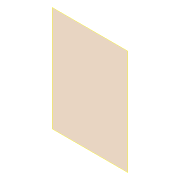
# Autodesk Inventor part: 30_Adapter_neje_LED
Saved by Autodesk Inventor 2019.4 (Build 234330000, 330)
## iProperties
Created: 2021-04-13
Part Number: 30_Adapter_neje_LED
Material: Generic
Document SubType Name: Modeling
Designer: diederichbenedict
Density: 1 g/cm^3
Appearance: Default
Author: diederichbenedict
Autodesk Inventor part; units mm, degrees
ref_plane "YZ Plane" through (0, 0, 0) normal (1, 0, 0) x (0, 1, 0)
ref_plane "XZ Plane" through (0, 0, 0) normal (0, 1, 0) x (-1, 0, 0)
ref_plane "XY Plane" through (0, 0, 0) normal (0, 0, 1) x (1, 0, 0)
ref_plane "Work Plane1" through (0, 0, 0) normal (0, 0, 1) x (1, 0, 0)
ref_plane "Work Plane2" through (0, 0, -24) normal (0, 0, 1) x (1, 0, 0)
sketch "Sketch1" plane through (0, 0, -24) normal (0, 0, 1) x (1, 0, 0)
  line L0 (-28.32, -15) -> (-28.32, -9.975) projected
  line L1 (-28.32, -3.975) -> (-28.32, 4.075) projected
  line L2 (-23.82, -15) -> (-28.32, -15) projected
  line L3 (-23.82, -15) -> (-23.52, -15)
  line L4 (-23.52, -15) -> (-23.82, -12.9669)
  line L5 (-23.82, -12.9669) -> (-18.8601, -12.9669)
  line L6 (-18.8601, -12.9669) -> (-18.8601, -18.9669)
  line L7 (-18.8601, -18.9669) -> (-92.6205, -18.9669)
  line L8 (-92.6205, -18.9669) -> (-92.6205, 137.182)
  line L9 (-92.6205, 137.182) -> (-83.4923, 137.182)
  line L10 (-83.4923, 137.182) -> (-83.4923, 6.5025)
  line L11 (-83.4923, 6.5025) -> (-28.32, 6.5025)
  line L12 (-28.32, -3.975) -> (-26.9128, -9.975)
  line L13 (-26.9128, -9.975) -> (-28.4348, -9.773)
  line L14 (-28.4348, -9.773) -> (-28.32, -10.5507)
  line L15 (-28.32, -10.5507) -> (-28.32, -15)
  line L16 (-28.32, -15) -> (-23.82, -15)
  line L17 (-28.32, 4.075) -> (-28.32, 4.2239)
  line L18 (-28.32, 4.2239) -> (-26.4709, 4.2239)
  line L19 (-26.4709, 4.2239) -> (-26.4709, 6.5025)
  line L20 (-26.4709, 6.5025) -> (-28.32, 6.5025)
  point P0 (0, 0)
  dimension "d0" = 0.3
  dimension "d1" = 6
  constraints: 36 end point, 9 perpendicular, 2 collinear, 2 parallel, 2 point on line, 1 horizontal, 1 vertical
  measures "d0" distance of L2.start L3.end
  measures "d1" distance of L5.end L6.end
extrude "Extrusion1" add sketch "Sketch1" along normal mid plane 20
fillet "Fillet1" radius 1 1 edges at (-26.9128, -9.975, -24)
chamfer "Chamfer1" distance 20 angle 45 2 edges at (-83.4923, 6.5025, -24) (-92.6205, -18.9669, -24)
sketch "Sketch2" plane through (-92.6205, 137.182, -34) normal (-1, 0, 0) x (0, 0, 1)
  line L0 (18.675, -27.877) -> (18.675, 6.063) projected
  line L1 (-16.4278, 9.4711) -> (-17.2496, 12.5384) projected
  line L2 (-17.2496, 12.5384) -> (-20.3169, 13.3602) projected
  line L3 (-20.3169, 13.3602) -> (-22.5622, 11.1149) projected
  line L4 (-22.5622, 11.1149) -> (-21.7404, 8.0476) projected
  line L5 (-21.7404, 8.0476) -> (-18.6731, 7.2258) projected
  line L6 (-18.6731, 7.2258) -> (-16.4278, 9.4711) projected
  line L7 (23.7269, -35.1742) -> (25.9722, -32.9289) projected
  line L8 (25.9722, -32.9289) -> (25.1504, -29.8616) projected
  line L9 (25.1504, -29.8616) -> (22.0831, -29.0398) projected
  line L10 (22.0831, -29.0398) -> (19.8378, -31.2851) projected
  line L11 (19.8378, -31.2851) -> (20.6596, -34.3524) projected
  line L12 (20.6596, -34.3524) -> (23.7269, -35.1742) projected
  circle A0 centre (16.005, 9.753) radius 2.475 projected
  circle A1 centre (-18.955, 3.393) radius 2.475 projected
  circle A2 centre (-12.595, -31.567) radius 2.475 projected
  circle A3 centre (22.365, -25.207) radius 2.475 projected
  circle A4 centre (22.365, 3.393) radius 2.475 projected
  circle A5 centre (16.005, -31.567) radius 2.475 projected
  circle A6 centre (-18.955, -25.207) radius 2.475 projected
  circle A7 centre (-12.595, 9.753) radius 2.475 projected
  arc A8 (-20.655, -19.707) -> (-17.255, -19.707) centre (-18.955, -19.707) ccw projected
  line L13 (-17.255, -19.707) -> (-17.255, -2.107) projected
  arc A9 (-17.255, -2.107) -> (-20.655, -2.107) centre (-18.955, -2.107) ccw projected
  line L14 (-20.655, -2.107) -> (-20.655, -19.707) projected
  arc A10 (20.665, -19.707) -> (24.065, -19.707) centre (22.365, -19.707) ccw projected
  line L15 (24.065, -19.707) -> (24.065, -2.107) projected
  arc A11 (24.065, -2.107) -> (20.665, -2.107) centre (22.365, -2.107) ccw projected
  line L16 (20.665, -2.107) -> (20.665, -19.707) projected
  arc A12 (10.505, -33.267) -> (10.505, -29.867) centre (10.505, -31.567) ccw projected
  line L17 (10.505, -29.867) -> (-7.095, -29.867) projected
  arc A13 (-7.095, -29.867) -> (-7.095, -33.267) centre (-7.095, -31.567) ccw projected
  line L18 (-7.095, -33.267) -> (10.505, -33.267) projected
  arc A14 (-7.095, 11.453) -> (-7.095, 8.053) centre (-7.095, 9.753) ccw projected
  line L19 (-7.095, 8.053) -> (10.505, 8.053) projected
  arc A15 (10.505, 8.053) -> (10.505, 11.453) centre (10.505, 9.753) ccw projected
  line L20 (10.505, 11.453) -> (-7.095, 11.453) projected
  line L21 (-15.265, -27.877) -> (18.675, -27.877) projected
  line L22 (18.675, -27.877) -> (18.675, 6.063) projected
  line L23 (18.675, 6.063) -> (-15.265, 6.063) projected
  line L24 (-15.265, 6.063) -> (-15.265, -27.877) projected
  circle A16 centre (-19.495, -32.107) radius 2.75 projected
  circle A17 centre (22.905, 10.293) radius 2.75 projected
  arc A18 (-22.645, -33.757) -> (-21.145, -35.257) centre (-21.145, -33.757) ccw projected
  line L25 (-22.645, 11.943) -> (-22.645, -33.757) projected
  arc A19 (-21.145, 13.443) -> (-22.645, 11.943) centre (-21.145, 11.943) ccw projected
  line L26 (24.555, 13.443) -> (-21.145, 13.443) projected
  arc A20 (26.055, 11.943) -> (24.555, 13.443) centre (24.555, 11.943) ccw projected
  line L27 (26.055, -33.757) -> (26.055, 11.943) projected
  arc A21 (24.555, -35.257) -> (26.055, -33.757) centre (24.555, -33.757) ccw projected
  line L28 (-21.145, -35.257) -> (24.555, -35.257) projected
  circle A22 centre (1.705, -10.907) radius 16.97
  circle A23 centre (15, -10.907) radius 2.65
  line L29 (20, 0) -> (20, -136.1489) projected
  line L30 (20, -136.1489) -> (0, -136.1489) projected
  line L31 (20, 0) -> (20, -136.1489) projected
  line L32 (0, 0) -> (20, 0) projected
  line L33 (0, -136.1489) -> (0, 0) projected
  line L34 (0, 0) -> (20, 0) projected
  line L35 (10, 0) -> (0, -136.1489)
  point P0 (34, -137.182)
  dimension "d8" = 5.3
  dimension "d9" = 5
  constraints: 3 tangent, 2 centre point, 2 end point, 1 midpoint
  measures "d8" diameter of A23
  measures "d9" distance from line of L29 A23.centre
extrude "Extrusion2" cut sketch "Sketch2" against normal through all contours L35 L17 L33 L21 | L21 A22 L35 | A22 L33 L32 L35 | L21 L33 A22 | L35 L18 L33 L17 | L35 L28 L33 L18 | L35 L33 L28 | A23
body "Solid1"
